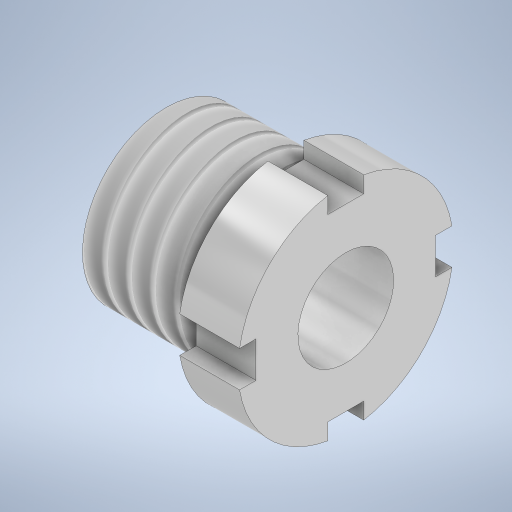
# Autodesk Inventor part: pieza 1-28
Saved by Autodesk Inventor 2024 (Build 280153000, 153)
## iProperties
Created: 2024-10-05
Part Number: pieza 1-28
Material: Aluminum 6061-AHC
Document SubType Name: Modeling
Designer: katam
Density: 2.7 g/cm^3
Appearance: Aluminum - Dark
Author: katam
Autodesk Inventor part; units mm, degrees
ref_plane "YZ Plane" through (0, 0, 0) normal (1, 0, 0) x (0, 1, 0)
ref_plane "XZ Plane" through (0, 0, 0) normal (0, 1, 0) x (-1, 0, 0)
ref_plane "XY Plane" through (0, 0, 0) normal (0, 0, 1) x (1, 0, 0)
sketch "Sketch1" plane through (0, 0, 0) normal (0, 0, 1) x (1, 0, 0)
  line L0 (0, 0) -> (0, 7) construction
  line L1 (0, 7) -> (10, 7)
  line L2 (0, 7) -> (1.5, 5.5)
  line L3 (10, 7) -> (10, 9)
  line L4 (10, 9) -> (15, 9)
  line L5 (15, 9) -> (15, 5.5)
  line L6 (15, 5.5) -> (1.5, 5.5)
  line L7 (0, 0) -> (19.3515, 0)
  line L8 (2, 4) -> (15, 4)
  line L9 (15, 4) -> (15, 5.5)
  line L10 (1.5, 5.5) -> (1.5, 0) construction
  line L11 (2, 5) -> (2, 4)
  line L12 (2, 5) -> (1.5, 5.5)
  dimension "d0" = 10
  dimension "d1" = 5
  dimension "d2" = 14
  dimension "d3" = 11
  dimension "d4" = 18
  dimension "d8" = 13
  dimension "d9" = 8
  dimension "d10" = 0.5
  constraints: 26 end point, 6 perpendicular, 2 point on line, 2 vertical, 1 horizontal
  measures "d0" distance of L0.end L1.end
  measures "d1" distance of L3.end L4.end
  measures "d2" diameter of L1 L7
  measures "d3" diameter of L6 L7
  measures "d4" diameter of L4 L7
  measures "d8" distance of L8.start L8.end
  measures "d9" diameter of L8 L7
  measures "d10" distance from line of L6 L11.start
revolve "Revolution1" add sketch "Sketch1" angle 360 about axis through (0, 0, 0) along (1, 0, 0)
sketch "Sketch2" plane through (15, 0, 0) normal (1, 0, 0) x (0, 0, -1)
  line L0 (-1.5, 9.5651) -> (1.5, 9.5651)
  line L1 (1.5, 9.5651) -> (1.5, 7.5)
  line L2 (1.5, 7.5) -> (-1.5, 7.5)
  line L3 (-1.5, 7.5) -> (-1.5, 9.5651)
  line L4 (8.9736, 1.4966) -> (8.9736, -0.0034)
  line L5 (7.5, -0.0034) -> (7.5, 1.4966)
  line L6 (-1.5, -7.5) -> (1.5, -7.5)
  line L7 (1.5, -7.5) -> (1.5, -9.612)
  line L8 (1.5, -9.612) -> (-1.5, -9.612)
  line L9 (-1.5, -9.612) -> (-1.5, -7.5)
  circle A0 centre (0, 0) radius 7 projected
  circle A1 centre (0, 0) radius 9 projected
  circle A2 centre (0, 0) radius 4 projected
  line L10 (7.2867, -0.0034) -> (9.9612, -0.0034) construction
  line L11 (7.5, 1.4966) -> (9, 1.4966)
  line L12 (7.5, -1.5034) -> (9, -1.5034)
  line L13 (7.5, -0.0034) -> (7.5, -1.5034)
  line L14 (9, 0) -> (9, -1.5034)
  line L15 (-10.5, 1.5) -> (-7.5, 1.5)
  line L16 (-7.5, 1.5) -> (-7.5, -1.5)
  line L17 (-7.5, -1.5) -> (-10.5, -1.5)
  line L18 (-10.5, -1.5) -> (-10.5, 1.5)
  line L19 (-10.5, 1.5) -> (-7.5, -1.5) construction
  line L20 (-7.5, 1.5) -> (-10.5, -1.5) construction
  point P0 (0, 9)
  point P1 (0, -9)
  point P2 (-9, 0)
  point P3 (-1.5, -8.8741)
  point P4 (1.5, -8.8741)
  point P5 (-8.8741, 1.5)
  point P6 (-8.8741, -1.5)
  point P7 (1.5, 8.8741)
  point P8 (-1.5, 8.8741)
  point P9 (8.8736, -1.5034)
  point P10 (8.8747, 1.4966)
  dimension "d11" = 1.5
  dimension "d12" = 1.5
  dimension "d13" = 1.5
  dimension "d16" = 1.5
  dimension "d18" = 1.5
  dimension "d20" = 3
  dimension "d21" = 3
  dimension "d22" = 3
  dimension "d23" = 1.5
  dimension "d24" = 3
  dimension "d25" = 1.5
  constraints: 42 end point, 7 parallel, 6 horizontal, 4 point on circle, 3 perpendicular, 3 point on line, 2 midpoint, 1 tangent, 1 vertical
  measures "d11" distance from line of A1.start L2
  measures "d12" distance from line of L5 L14.start
  measures "d13" distance from line of L6 point (0, -9)
  measures "d16" distance between parallel lines of L11 L10
  measures "d18" distance between parallel lines of L10 L12
  measures "d20" distance of L16.end L17.end
  measures "d21" distance between parallel lines of L17 L15
  measures "d22" distance of L1.end L2.end
  measures "d23" distance from line of A1.start L1
  measures "d24" distance of L6.start L6.end
  measures "d25" distance from line of point (0, -9) L7
extrude "Extrusion1" cut sketch "Sketch2" against normal blind 10 contours A1 L1 L2 L3 | L15 L16 L17 A1 | A1 L12 L13 L5 L11 | L9 L6 L7 A1
thread "Thread1" size "M14x2" class "6g" standard "ANSI Metric M Profile" length 24.5
body "Solid1"
